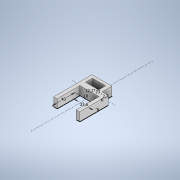
# Autodesk Inventor part: LegEnd_v1
Saved by Autodesk Inventor 2020.3 (Build 243373000, 373)
## iProperties
Created: 2021-02-26
Part Number: LegEnd_v1
Material: Generic
Document SubType Name: Modeling
Designer: sanyi
Density: 1 g/cm^3
Appearance: Default
Author: sanyi
Autodesk Inventor part; units mm, degrees
ref_plane "YZ Plane" through (0, 0, 0) normal (1, 0, 0) x (0, 1, 0)
ref_plane "XZ Plane" through (0, 0, 0) normal (0, 1, 0) x (-1, 0, 0)
ref_plane "XY Plane" through (0, 0, 0) normal (0, 0, 1) x (1, 0, 0)
sketch "Sketch1" plane through (0, 0, 0) normal (0, 1, 0) x (-1, 0, 0)
  line L0 (0, 114.4425) -> (0, 11.1) construction
  line L1 (41.9698, 0) -> (-35.0855, 0) construction
  line L2 (-11.5, 6.1) -> (11.5, 6.1)
  line L3 (11.5, 6.1) -> (11.5, -6.1)
  line L4 (11.5, -6.1) -> (-11.5, -6.1)
  line L5 (-11.5, -6.1) -> (-11.5, 6.1)
  line L6 (-17.5, -11.1) -> (17.5, -11.1)
  line L7 (11.5, 16.1) -> (11.5, 56.1)
  line L8 (11.5, 56.1) -> (17.5, 56.1)
  line L9 (11.5, 16.1) -> (-17.5, 16.1)
  line L10 (17.5, 56.1) -> (17.5, -11.1)
  line L11 (-17.5, 6.1) -> (-28.1, 6.1)
  line L12 (-17.5, 16.1) -> (-22.1, 16.1)
  line L13 (-22.1, 16.1) -> (-22.1, 56.1)
  line L14 (-22.1, 56.1) -> (-28.1, 56.1)
  line L15 (-28.1, 56.1) -> (-28.1, 6.1)
  line L16 (-17.5, 6.1) -> (-17.5, -11.1)
  line L17 (11.5, -6.1) -> (11.5, -11.1)
  line L18 (0, -6.1) -> (0, -11.1)
  line L19 (0, -11.1) -> (0, -101.7) construction
  line L20 (11.5, 6.1) -> (11.5, 11.1)
  line L21 (11.5, 11.1) -> (0, 11.1)
  line L22 (0, 6.1) -> (0, -6.1) construction
  line L23 (0, 11.1) -> (0, 6.1)
  point P0 (0, 0)
  point P1 (14.2, 0)
  point P2 (-14.2, 0)
  dimension "d4" = 23
  dimension "d5" = 12.2
  dimension "d8" = 2.7
  dimension "d9" = 5
  dimension "d11" = 10
  dimension "d12" = 40
  dimension "d14" = 33.6
  dimension "d15" = 6
  dimension "d16" = 6
  constraints: 48 end point, 9 perpendicular, 7 vertical, 5 horizontal, 5 point on line, 4 midpoint, 3 collinear, 3 parallel, 1 symmetric about line, 4 other
  measures "d4" distance of L3.end L4.end
  measures "d5" distance of L2.end L3.end
  measures "d8" distance from line of L5 point (-14.2, 0)
  measures "d9" distance between parallel lines of L6 L4
  measures "d11" distance between parallel lines of L2 L9
  measures "d12" distance between parallel lines of L9 L8
  measures "d14" distance between parallel lines of L13 L7
  measures "d15" distance between parallel lines of L16 L5
  measures "d16" distance between parallel lines of L15 L13
extrude "Extrusion1" add sketch "Sketch1" along normal blind 15 contours L5 L4 L18 L6 L16 L11 L15 L14 L13 L12 L9 L7 L8 L10 L17 L3 L20 L21 L23 L2 | L23 L21 L20 L2 | L4 L17 L6 L18
body "Solid1"
